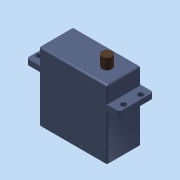
# Autodesk Inventor part: servo20kg-ds8120
Saved by Autodesk Inventor 2015 SP1 (Build 190203100, 203)
## iProperties
Created: 2023-12-10
Part Number: servo20kg-ds8120
Material: Типовые
Document SubType Name: Modeling
Designer: boss
Density: 1 g/cm^3
Appearance: По умолчанию
Author: boss
Autodesk Inventor part; units mm, degrees
ref_plane "YZ Plane" through (0, 0, 0) normal (1, 0, 0) x (0, 1, 0)
ref_plane "XZ Plane" through (0, 0, 0) normal (0, 1, 0) x (-1, 0, 0)
ref_plane "XY Plane" through (0, 0, 0) normal (0, 0, 1) x (1, 0, 0)
sketch "Эскиз1" plane through (0, 0, 0) normal (0, 0, 1) x (1, 0, 0)
  line L0 (-25.75, 10) -> (25.75, 10)
  line L1 (27.25, 8.5) -> (27.25, -8.5)
  line L2 (25.75, -10) -> (-25.75, -10)
  line L3 (-27.25, -8.5) -> (-27.25, 8.5)
  line L4 (-27.25, 10) -> (27.25, -10) construction
  line L5 (27.25, 10) -> (-27.25, -10) construction
  line L6 (-20, 10) -> (20, 10)
  line L7 (20, 10) -> (20, -10)
  line L8 (20, -10) -> (-20, -10)
  line L9 (-20, -10) -> (-20, 10)
  line L10 (-20, 10) -> (20, -10) construction
  line L11 (20, 10) -> (-20, -10) construction
  arc A0 (27.25, 8.5) -> (25.75, 10) centre (25.75, 8.5) ccw
  arc A1 (25.75, -10) -> (27.25, -8.5) centre (25.75, -8.5) ccw
  arc A2 (-27.25, -8.5) -> (-25.75, -10) centre (-25.75, -8.5) ccw
  arc A3 (-25.75, 10) -> (-27.25, 8.5) centre (-25.75, 8.5) ccw
  line L12 (-34.7079, 0) -> (34.7079, 0) construction
  circle A4 centre (10, 0) radius 2.95
  line L13 (24.75, -5) -> (-24.75, -5) construction
  line L14 (-24.75, -5) -> (-24.75, 5) construction
  line L15 (-24.75, 5) -> (24.75, 5) construction
  line L16 (24.75, 5) -> (24.75, -5) construction
  line L17 (24.75, -5) -> (-24.75, 5) construction
  line L18 (-24.75, -5) -> (24.75, 5) construction
  circle A5 centre (-24.75, 5) radius 1.6
  circle A6 centre (-24.75, -5) radius 1.6
  circle A7 centre (24.75, 5) radius 1.6
  circle A8 centre (24.75, -5) radius 1.6
  point P0 (0, 0)
  point P1 (0, 0)
  dimension "d0" = 54.5
  dimension "d1" = 20
  dimension "d2" = 40
  dimension "d3" = 20
  dimension "d4" = 1.5
  dimension "d5" = 5.9
  dimension "d6" = 10
  dimension "d7" = 49.5
  dimension "d8" = 10
  dimension "d9" = 3.2
  dimension "d10" = 3.2
  dimension "d11" = 3.2
  dimension "d12" = 3.2
  dimension "d22" = 17.25
  constraints: 38 end point, 9 centre point, 9 point on line, 8 midpoint, 8 point on circle, 8 tangent, 6 parallel, 4 coincident, 4 horizontal, 3 equal radius, 3 perpendicular
  measures "d0" distance of L4.end L5.end
  measures "d1" distance of L5.start L4.end
  measures "d2" distance of L7.end L8.end
  measures "d3" distance of L6.end L7.end
  measures "d4" radius of A0
  measures "d5" diameter of A4
  measures "d6" distance from line of L7 A4.centre
  measures "d7" distance of L14.end L15.end
  measures "d8" distance of L13.end L14.end
  measures "d9" diameter of A5
  measures "d10" diameter of A6
  measures "d11" diameter of A7
  measures "d12" diameter of A8
  measures "d22" horizontal distance of L1.start A4.centre
extrude "Выдавливание1" add sketch "Эскиз1" along normal blind 12.7 and the other way blind 27.8 contours L0 L7 L2 L9 | A4
extrude "Выдавливание2" add sketch "Эскиз1" along normal blind 18.9 separate body contours A4
extrude "Выдавливание3" add sketch "Эскиз1" along normal blind 3.1 contours L0 L9 L2 A2 L3 A3 | L0 A0 L1 A1 L2 L7 bodies 1
fillet "Сопряжение1" radius 1 16 edges at (20, 10, -13.9) (0, 10, -27.8) (20, 0, -27.8) (20, -10, -13.9) (20, 0, 12.7) (20, 10, 7.9) (0, -10, -27.8) (-20, 10, -13.9) (-20, 0, -27.8) (-20, 10, 7.9) (-20, 0, 12.7) (-20, -10, 7.9) (0, -10, 12.7) (0, 10, 12.7) (20, -10, 7.9) (-20, -10, -13.9)
equation "\"servaBodyHeght\" = 40.5"
